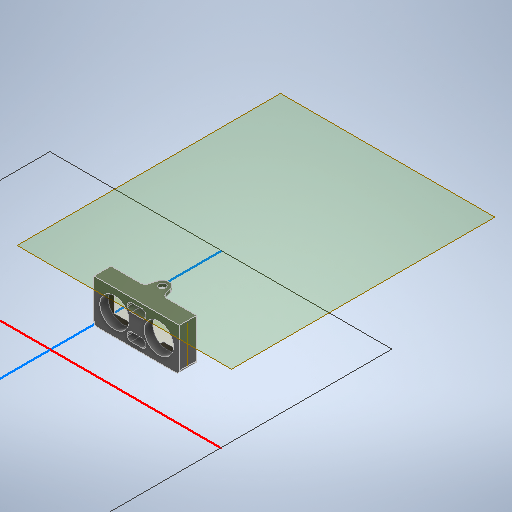
# Autodesk Inventor part: suporte ultrasom
Saved by Autodesk Inventor 2025.1 (Build 291241000, 241)
## iProperties
Created: 2024-09-06
Part Number: suporte ultrasom
Material: Genérico
Document SubType Name: Modeling
Designer: Célio
Density: 1 g/cm^3
Appearance: Suave - Preto
Author: Célio
Autodesk Inventor part; units mm, degrees
ref_plane "YZ Plane" through (0, 0, 0) normal (1, 0, 0) x (0, 1, 0)
ref_plane "XZ Plane" through (0, 0, 0) normal (0, 1, 0) x (-1, 0, 0)
ref_plane "XY Plane" through (0, 0, 0) normal (0, 0, 1) x (1, 0, 0)
ref_plane "Plano de trabalho1" through (25.8382, -7.4236, -29.9034) normal (0, 0, 1) x (1, 0, 0)
sketch "Esboço1" plane through (25.8382, -7.4236, -29.9034) normal (0, 0, 1) x (1, 0, 0)
  line L0 (-23, 10.5) -> (23, 10.5)
  line L1 (23, 10.5) -> (23, -10.5)
  line L2 (23, -10.5) -> (-23, -10.5)
  line L3 (-23, -10.5) -> (-23, 10.5)
  line L4 (23, 12.5) -> (-23, 12.5)
  line L5 (-25, 10.5) -> (-25, -10.5)
  line L6 (-23, -12.5) -> (23, -12.5)
  line L7 (25, -10.5) -> (25, 10.5)
  arc A0 (23, -12.5) -> (25, -10.5) centre (23, -10.5) ccw
  arc A1 (-25, -10.5) -> (-23, -12.5) centre (-23, -10.5) ccw
  circle A2 centre (-13, 0) radius 8.5
  circle A3 centre (13, 0) radius 8.5
  line L8 (-23, 10.5) -> (23, -10.5) construction
  line L9 (23, 10.5) -> (-23, -10.5) construction
  line L10 (-3.25, 4.9) -> (3.25, 4.9)
  line L11 (5.25, 6.9) -> (5.25, 7.9)
  line L12 (3.25, 9.9) -> (-3.25, 9.9)
  line L13 (-5.25, 7.9) -> (-5.25, 6.9)
  line L14 (-5.25, 4.9) -> (5.25, 9.9) construction
  line L15 (5.25, 4.9) -> (-5.25, 9.9) construction
  arc A4 (-3.25, 9.9) -> (-5.25, 7.9) centre (-3.25, 7.9) ccw
  arc A5 (-5.25, 6.9) -> (-3.25, 4.9) centre (-3.25, 6.9) ccw
  arc A6 (3.25, 4.9) -> (5.25, 6.9) centre (3.25, 6.9) ccw
  arc A7 (5.25, 7.9) -> (3.25, 9.9) centre (3.25, 7.9) ccw
  line L16 (0, 0) -> (0, -7.4)
  line L17 (-3.25, -9.9) -> (3.25, -9.9)
  line L18 (5.25, -7.9) -> (5.25, -6.9)
  line L19 (3.25, -4.9) -> (-3.25, -4.9)
  line L20 (-5.25, -6.9) -> (-5.25, -7.9)
  line L21 (-5.25, -9.9) -> (5.25, -4.9) construction
  line L22 (5.25, -9.9) -> (-5.25, -4.9) construction
  arc A8 (-3.25, -4.9) -> (-5.25, -6.9) centre (-3.25, -6.9) ccw
  arc A9 (-5.25, -7.9) -> (-3.25, -9.9) centre (-3.25, -7.9) ccw
  arc A10 (3.25, -9.9) -> (5.25, -7.9) centre (3.25, -7.9) ccw
  arc A11 (5.25, -6.9) -> (3.25, -4.9) centre (3.25, -6.9) ccw
  line L23 (-23, 12.5) -> (-25, 12.5)
  line L24 (-25, 12.5) -> (-25, 10.5)
  line L25 (23, 12.5) -> (25, 12.5)
  line L26 (25, 12.5) -> (25, 10.5)
  point P0 (-25.8382, 7.4236)
  dimension "d0" = 2
  dimension "d4" = 46
  dimension "d5" = 21
  dimension "d7" = 17
  dimension "d9" = 17
  dimension "d16" = 7.4
  constraints: 54 end point, 20 point on circle, 20 tangent, 18 point on line, 12 centre point, 8 parallel, 6 equal radius, 6 perpendicular, 4 horizontal, 1 midpoint, 1 vertical, 3 other
  measures "d0" distance between parallel lines of L0 L4
  measures "d4" distance of L0.start L0.end
  measures "d5" distance of L0.end L1.end
  measures "d7" diameter of A2
  measures "d9" diameter of A3
  measures "d16" distance of L16.start L16.end
extrude "Extrusão1" add sketch "Esboço1" along normal blind 5 contours L0 L1 L2 L3 | L25 L26 L7 A0 L6 A1 L5 L24 L23 L4
extrude "Extrusão2" add sketch "Esboço1" against normal blind 5 contours L25 L26 L7 A0 L6 A1 L5 L24 L23 L4
sketch "Esboço2" plane through (2.8382, -19.9236, -24.9034) normal (0, -1, 0) x (1, 0, 0)
  line L0 (28.5, -9.5) -> (28.5, -7.75)
  line L1 (28.5, -7.75) -> (17.5, -7.75)
  line L2 (17.5, -7.75) -> (17.5, -9.5)
  line L3 (46, -10) -> (0, -10) projected
  line L4 (17.5, -10) -> (28.5, -10)
  line L5 (23, -12) -> (31, -12)
  line L6 (23, -12) -> (15, -12)
  line L7 (15, -12) -> (15, -10)
  line L8 (17, -10) -> (15, -10)
  line L9 (31, -12) -> (31, -10)
  line L10 (29, -10) -> (31, -10)
  arc A0 (28.5, -9.5) -> (29, -10) centre (29, -9.5) ccw
  arc A1 (17, -10) -> (17.5, -9.5) centre (17, -9.5) ccw
  point P0 (-2.8382, 24.9034)
  point P1 (23, -10)
  point P2 (17, -10)
  dimension "d24" = 8
  dimension "d25" = 8
  dimension "d26" = 0.5
  dimension "d27" = 0.5
  constraints: 20 end point, 8 point on line, 4 point on circle, 4 tangent, 2 centre point, 2 collinear, 2 horizontal, 2 perpendicular, 1 midpoint, 1 parallel
  measures "d24" distance of L5.start L5.end
  measures "d25" distance of L5.start L6.end
  measures "d26" radius of A0
  measures "d27" radius of A1
extrude "Extrusão3" cut sketch "Esboço2" against normal up to surface (2 mm away) contours A0 L3 A1 L2 L1 L0
ref_plane "Plano de trabalho2" through (25.638, 5.0764, -94.896) normal (0, -1, 0) x (0, 0, 1)
sketch "Esboço5" plane through (0.8382, 5.0764, -24.9034) normal (0, 1, 0) x (1, 0, 0)
  line L0 (48, 10) -> (2, 10) projected
  circle A0 centre (25, 15) radius 2
  arc A1 (28.8606, 16.0467) -> (21.1394, 16.0467) centre (25, 15) ccw
  line L1 (19.5, 10) -> (21.1394, 16.0467)
  line L2 (30.5, 10) -> (28.8606, 16.0467)
  line L3 (30.5, 10) -> (19.5, 10)
  line L4 (0, 10) -> (50, 10) projected
  point P0 (-0.8382, -24.9034)
  dimension "d56" = 4
  dimension "d57" = 2
  constraints: 6 end point, 2 centre point, 2 point on circle, 2 point on line, 2 tangent, 1 collinear
  measures "d56" diameter of A0
  measures "d57" radial gap between concentric circles of A0 A1
extrude "Extrusão5" add sketch "Esboço5" against normal blind 2
fillet "Arredondamento3" radius 3 2 edges at (20.3382, 4.0764, -34.9034) (31.3382, 4.0764, -34.9034)
